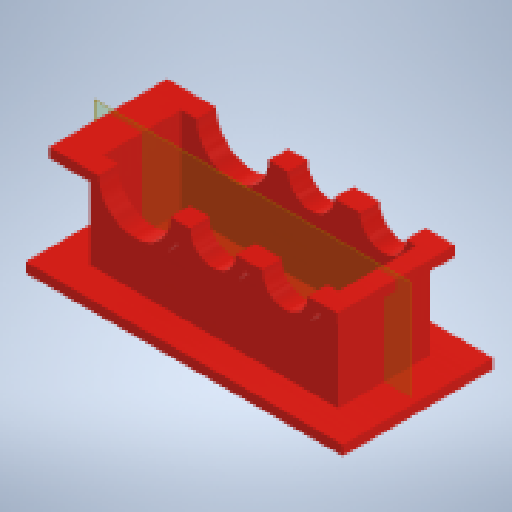
# Autodesk Inventor part: Part8
Saved by Autodesk Inventor 2023 (Build 270158000, 158)
## iProperties
Created: 2023-01-29
Part Number: Part8
Material: Generic
Document SubType Name: Modeling
Designer: Merve Babacan
Density: 1 g/cm^3
Appearance: Orange-Red
Author: Merve Babacan
Autodesk Inventor part; units mm, degrees
ref_plane "YZ Plane" through (0, 0, 0) normal (1, 0, 0) x (0, 1, 0)
ref_plane "XZ Plane" through (0, 0, 0) normal (0, 1, 0) x (-1, 0, 0)
ref_plane "XY Plane" through (0, 0, 0) normal (0, 0, 1) x (1, 0, 0)
sketch "Sketch1" plane through (0, 0, 0) normal (0, 0, 1) x (1, 0, 0)
  arc A0 (-55, 0) -> (55, 0) centre (0, 0) ccw
  arc A1 (-70, 0) -> (63.2456, -30) centre (0, 0) ccw
  arc A2 (85, 0) -> (155, 0) centre (120, 0) ccw
  arc A3 (80, -30) -> (167.697, -15) centre (120, 0) ccw
  arc A4 (195, 0) -> (265, 0) centre (230, 0) ccw
  arc A5 (182.303, -15) -> (277.697, -15) centre (230, 0) ccw
  line L0 (-130, 0) -> (-130, -15)
  line L1 (310, -15) -> (310, 0)
  line L2 (-130, -15) -> (-68.374, -15)
  line L3 (-130, 0) -> (-55, 0)
  line L4 (63.2456, -30) -> (80, -30)
  line L5 (167.697, -15) -> (182.303, -15)
  line L6 (277.697, -15) -> (310, -15)
  line L7 (265, 0) -> (310, 0)
  line L8 (55, 0) -> (85, 0)
  line L9 (155, 0) -> (195, 0)
  line L10 (-88.374, -15) -> (-88.374, -145)
  line L11 (-88.374, -145) -> (291.626, -145)
  line L12 (291.626, -145) -> (291.626, -15)
  dimension "d0" = 110
  dimension "d1" = 140
  dimension "d2" = 70
  dimension "d3" = 100
  dimension "d4" = 70
  dimension "d5" = 100
  dimension "d8" = 440
  dimension "d9" = 130
  dimension "d10" = 15
  dimension "d12" = 130
  dimension "d13" = 380
  dimension "d14" = 20
  constraints: 26 end point, 13 point on circle, 6 centre point, 5 perpendicular, 4 coincident, 4 horizontal, 3 point on line, 2 vertical
  measures "d0" diameter of A0
  measures "d1" diameter of A1
  measures "d2" diameter of A2
  measures "d3" diameter of A3
  measures "d4" diameter of A4
  measures "d5" diameter of A5
  measures "d8" distance of L0.start L1.end
  measures "d9" distance of L0.start point (0, 0)
  measures "d10" distance of L0.start L0.end
  measures "d12" distance of L10.start L10.end
  measures "d13" distance of L10.end L11.end
  measures "d14" distance of L2.end L10.start
extrude "Extrusion1" add sketch "Sketch1" along normal blind 30 contours A0 L8 A2 L9 A4 L7 L1 L6 A5 L5 A3 L4 A1 L3 | A1 L2 L0 L3
extrude "Extrusion2" add sketch "Sketch1" along normal blind 10 contours A1 L4 A3 L5 A5 L6 L12 L11 L10 L2
sketch "Sketch2" plane through (0, 0, 0) normal (0, 0, -1) x (-1, 0, 0)
  line L0 (-291.626, -145) -> (-291.626, -15) projected
  line L1 (88.374, -145) -> (-291.626, -145) projected
  line L2 (88.374, -15) -> (88.374, -145) projected
  line L3 (-281.626, -15) -> (-281.626, -135)
  line L4 (-281.626, -135) -> (78.374, -135)
  line L5 (78.374, -135) -> (78.374, -15)
  line L6 (-291.626, -15) -> (-310, -15) projected
  line L7 (130, -15) -> (88.374, -15) projected
  line L8 (-291.626, -15) -> (-281.626, -15)
  line L9 (78.374, -15) -> (88.374, -15)
  point P0 (0, 0)
  dimension "d19" = 10
  constraints: 10 end point, 2 horizontal, 2 other
  measures "d19" distance between parallel lines of L1 L4
extrude "Extrusion3" add sketch "Sketch2" along normal blind 130
ref_plane "Work Plane1" through (0, 0, -60) normal (0, 0, -1) x (-1, 0, 0)
mirror "Mirror1" about plane through (0, 0, -60) normal (0, 0, -1) of "Extrusion1", "Extrusion2"
sketch "Sketch3" plane through (0, 0, -60) normal (0, 0, -1) x (-1, 0, 0)
  line L0 (78.374, -135) -> (78.374, -15) projected
  line L1 (130, 0) -> (130, -15) projected
  line L2 (78.374, -15) -> (130, -15)
  line L3 (130, -15) -> (130, 0)
  line L4 (130, 0) -> (78.374, 0)
  line L5 (78.374, 0) -> (78.374, -15)
  line L6 (-281.626, -15) -> (-281.626, -135) projected
  line L7 (-310, 0) -> (-265, 0) projected
  line L8 (-281.626, -15) -> (-310, -15)
  line L9 (-310, -15) -> (-310, 0)
  line L10 (-310, 0) -> (-281.626, 0)
  line L11 (-281.626, 0) -> (-281.626, -15)
  point P0 (0, 0)
  constraints: 16 end point, 4 parallel, 2 horizontal, 2 perpendicular
extrude "Extrusion4" add sketch "Sketch3" along normal through all both and the other way through all
sketch "Sketch4" plane through (0, 0, -60) normal (0, 0, -1) x (-1, 0, 0)
  line L0 (-291.626, -15) -> (-291.626, -145) projected
  line L1 (-343.586, -145) -> (141.414, -145)
  line L2 (141.414, -145) -> (141.414, -160)
  line L3 (141.414, -160) -> (-343.586, -160)
  line L4 (-343.586, -145) -> (-343.586, -160)
  point P0 (0, 0)
  dimension "d29" = 51.96
  dimension "d30" = 485
  dimension "d31" = 15
  constraints: 8 end point, 2 horizontal, 1 parallel, 1 perpendicular, 1 vertical
  measures "d29" distance from line of L0 L1.start
  measures "d30" distance of L2.end L3.end
  measures "d31" distance of L1.end L2.end
extrude "Extrusion5" add sketch "Sketch4" along normal mid plane 230
body "Solid1"
